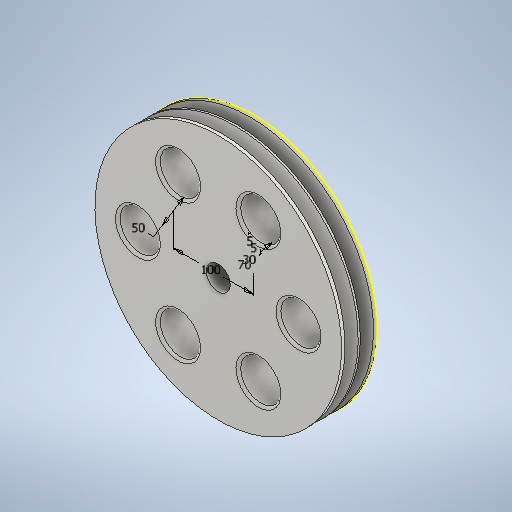
# Autodesk Inventor part: Grooved Pulley2
Saved by Autodesk Inventor 2025 (Build 290162000, 162)
## iProperties
CustomPartVersion: 1
Created: 2025-05-25
Part Number: Grooved Pulley2
Material: Steel
Document SubType Name: Modeling
Designer: Abdullah
Density: 1 g/cm^3
Appearance: Steel
Author: Abdullah
Autodesk Inventor part; units mm, degrees
ref_plane "YZ Plane" through (0, 0, 0) normal (1, 0, 0) x (0, 1, 0)
sketch "Main Sketch" plane through (0, 0, 0) normal (1, 0, 0) x (0, 1, 0)
  line L0 (0, 44) -> (153.5, 44)
  line L1 (153.5, 44) -> (153.5, 20.7051)
  line L2 (153.5, 20.7051) -> (136, 14.6794)
  line L3 (136, 14.6794) -> (136, 10.3206)
  line L4 (136, 10.3206) -> (153.5, 4.2949)
  line L5 (153.5, 4.2949) -> (153.5, 0)
  line L6 (153.5, 0) -> (0, 0)
  line L7 (150, 19.5) -> (150, 5.5) construction
  line L8 (136, 12.5) -> (150, 12.5) construction
  line L9 (153.5, 20.7051) -> (153.5, 4.2949)
  line L10 (0, -4) -> (0, 24) projected
  line L11 (0, 0) -> (0, 44)
  dimension "d0" = 14
  dimension "d1" = 38
  dimension "d2" = 3.5
  dimension "d6" = 44
  dimension "d21" = 300
  dimension "d25" = 17.5
  dimension "d27" = 12.5
  constraints: 22 end point, 5 perpendicular, 2 collinear, 2 midpoint, 2 point on line, 1 parallel
  measures "d0" distance of L7.start L7.end
  measures "d1" angle of L2 L4
  measures "d2" distance between parallel lines of L1 L7
  measures "d6" distance between parallel lines of L6 L0
  measures "d21" diameter of L7 L10
  measures "d25" distance between parallel lines of L3 L9
  measures "d27" distance between parallel lines of L6 L8
ref_plane "Belt Plane" through (0, 136, 12.5) normal (0, 0, 1) x (1, 0, 0)
revolve "Body" add sketch "Main Sketch" angle 360 about axis through (0, 0, -10) along (0, 0, 1)
revolve "Groove" cut sketch "Main Sketch" angle 360 about axis through (0, 0, -10) along (0, 0, 1) contours L9 L4 L3 L2
fillet "Fillet External" [suppressed]
fillet "Fillet Internal" [suppressed]
pattern_linear "Groove Pattern" count 2 spacing 19 along (0, 0, 1) of "Groove"
sketch "Sketch2" plane through (0, 0, 0) normal (0, 0, -1) x (-1, 0, 0)
  circle A0 centre (0, 0) radius 15
  circle A1 centre (0, 0) radius 35
  line L0 (-2.5, 17.5) -> (2.5, 17.5)
  line L1 (2.5, 17.5) -> (2.5, 12.5)
  line L2 (2.5, 12.5) -> (-2.5, 12.5)
  line L3 (-2.5, 12.5) -> (-2.5, 17.5)
  line L4 (-2.5, 17.5) -> (2.5, 12.5) construction
  line L5 (2.5, 17.5) -> (-2.5, 12.5) construction
  line L6 (0, 0) -> (153.5, 0)
  circle A2 centre (0, 0) radius 153.5 projected
  circle A3 centre (100, 0) radius 25
  point P0 (0, 15)
  point P1 (-2.5, 14.7902)
  point P2 (2.5, 14.7902)
  dimension "d28" = 30
  dimension "d29" = 70
  dimension "d30" = 5
  dimension "d31" = 5
  dimension "d44" = 50
  dimension "d45" = 100
  constraints: 14 end point, 2 centre point, 2 coincident, 2 horizontal, 2 midpoint, 2 parallel, 1 horizontal alignment, 1 perpendicular, 1 point on line, 4 other
  measures "d29" diameter of A1
  measures "d30" distance of L1.end L2.end
  measures "d31" distance of L0.end L1.end
  measures "d44" diameter of A3
  measures "d45" distance of point (0, 0) A3.centre
extrude "Extrusion1" cut sketch "Sketch2" against normal through all contours A0 L3 L2 L1 | L1 L2 L3 A0
extrude "Extrusion2" add sketch "Sketch2" along normal blind 50 contours A1
ref_plane "Work Plane2" through (0, 35, 0) normal (0, 1, 0) x (-1, 0, 0)
sketch "Sketch3" plane through (0, 35, 0) normal (0, 1, 0) x (-1, 0, 0)
  circle A0 centre (0, -23.9636) radius 4
  point P0 (0, 0)
  dimension "d36" = 8
  constraints: 1 centre point
  measures "d36" diameter of A0
extrude "Extrusion3" cut sketch "Sketch3" against normal blind 26.5
thread "Thread1" size "M8x1.25" class "6H" standard "ANSI Metric M Profile" full length
pattern_circular "Circular Pattern1" count 2 over 90 about axis through (0, 0, 0) along (0, 0, 1) of "Extrusion3"
extrude "Extrusion4" cut sketch "Sketch2" against normal through all contours A3 L6 | L6 A3
pattern_circular "Circular Pattern2" count 6 over 360 about axis through (0, 0, 0) along (0, 0, -1) of "Extrusion4"
fillet "Fillet3" radius 3 13 edges at (37.5, 64.9519, 0) (37.5, 64.9519, 44) (-37.5, 64.9519, 0) (-37.5, 64.9519, 44) (-75, 0, 0) (-75, 0, 44) (-37.5, -64.9519, 0) (-37.5, -64.9519, 44) (37.5, -64.9519, 0) (37.5, -64.9519, 44) (75, 0, 0) (75, 0, 44) (35, 0, 0)
equation "\"d0\" = da_Bw"
equation "\"d1\" = da_Alfa"
equation "\"d2\" = da_c"
equation "\"d21\" = da_Dw"
equation "\"d25\" = da_Hd"
equation "\"d27\" = da_Se"
equation "\"da_r1\" = 0"
equation "\"da_r2\" = 0"
equation "\"d18\" = da_Sg"
equation "\"d5\" = da_Se"
equation "\"da_Bw\" = 14"
equation "\"da_Alfa\" = 38deg"
equation "\"da_c\" = 3.5"
equation "\"da_Dw\" = 300"
equation "\"da_Hd\" = 17.5"
equation "\"da_Se\" = 12.5"
equation "\"da_Sg\" = 19"
body "Solid1"
